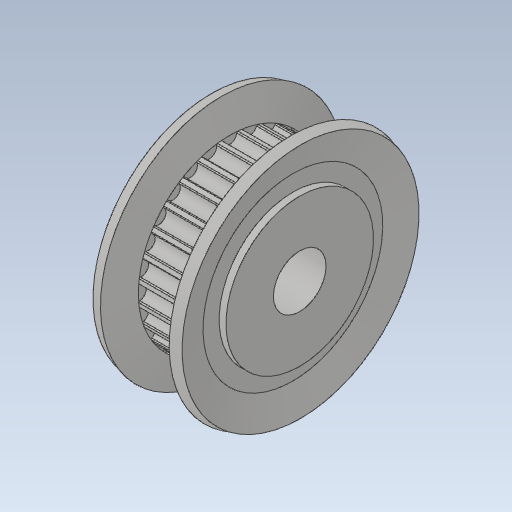
# Autodesk Inventor part: GPA28GT2040-A-H5_b
Saved by Autodesk Inventor 2024 (Build 280153000, 153)
## iProperties
Created: 2023-09-30
Part Number: GPA28GT2040-A-H5_b
Material: Generic
Catalog Web Link: www.cadenas.de
Description: GPA_GT2040, GPA_GT2060, GPA_GT2090, KGPA_GT2040, KGPA_GT2060, KGPA_GT2090, KGPK_GT2040, KGPK_GT2060, KGPK_GT2090_body-High Torque Timing Pulleys 2GT Type
Vendor: MISUMI
Document SubType Name: Modeling
Designer: psAdmin
Manufacturer: MISUMI
Mass: 1.92653 g
Surface Area: 18.9282 cm^2
Volume: 1.92653 cm^3
Density: 1 g/cm^3
Appearance: PSOLRGB-175-175-175
Category: PARTsolutions
Company: MISUMI
PSOL_IDENT_0: {$CADENAS_DATA/23d-libs/misumi/metric/51_timing_pulleys/gpa__gt2/gpa_gt2.prj},477 {VTYP=3D},{NB=GPA2
PSOL_IDENT_1: 8GT2040-A-H5_b},{LINA=GPA28GT2040-A-H5},{NN=GPA_GT2040, GPA_GT2060, GPA_GT2090, KGPA_GT2040, KGPA_GT
PSOL_IDENT_2: 2060, KGPA_GT2090, KGPK_GT2040, KGPK_GT2060, KGPK_GT2090_body},{DATE=25.04.2022 01:22:58},{GEOMDATE=
PSOL_IDENT_3: 22.12.2021 00:45:33},{VERSION=},{LINEID=100},{WBVAR=MAT,ST,TNW,PS,SBS,DD,Z,J,Q,R,S,T,ALT1,ALT2,M,QSC
PSOL_IDENT_4: ,QFC,QTC,ALT3,K,KSC,KFC,KTC,ALT4,ZM,ZSC,ZFC,ZTC,ALT5,BC,ALT6,ALT7,ALT8,FC,ALT13,BN},{WBNUMERIC=DD,Z,
PSOL_IDENT_5: J,Q,R,S,T,QSC,QFC,QTC,K,KSC,KFC,KTC,ZSC,ZFC,ZTC,BC,FC,BN}  {NB=GPA28GT2040-A-H5_b},{LINA=GPA28GT2040
PSOL_IDENT_6: -A-H5},{KT=DUMMY},{PN=GPA28GT2040-A-H5},{TYPE=GPA},{MAT=AA},{ST=CA},{NT=28},{TNW=GT2040},{BW=0},{A=5
PSOL_IDENT_7: .0},{W=8.3},{L=16.0},{PS=A},{PSA= 'A','B' },{SBS=H},{SBSALG= 'H','Round Hole','V','Stepped Hole' },{
PSOL_IDENT_8: DD=5.00},{DDALG=[5:6/1],[6.35],[7:10/1]},{DDHA=[5:6/1],[6.35],[7:10/1]},{DDHB=[5:6/1],[6.35],[7:8/1]
PSOL_IDENT_9: },{DDPA=},{DDPB=},{DDNA=},{DDNB=},{DDNKA=0},{DDNKB=0},{DDVA=[5:6/1],[6.35],[7:8/1]},{DDVFB=},{DDYA=[
PSOL_IDENT_10: 5:8/1]},{Z=0},{ZALG=0},{ZMIN=7},{ZAMAX=10},{ZBMAX=0},{J=0.0},{JALG=0},{JMAX=6.3},{Q=0},{R=0},{QRALG=
PSOL_IDENT_11: 0},{QRMIN=7},{QRMAX=10},{S=0.0},{SALG=0},{SMAX=2.300},{T=0.0},{TALG=0},{TMAX=5.000},{PD=17.83},{OD=1
PSOL_IDENT_12: 7.32},{D=10},{DE=14},{DDZ=5},{F=23},{E=14},{BB=0},{TT=0},{M1=3},{AC=-},{ALT1=},{ALT1A= '','Not appli
PSOL_IDENT_13: cable' },{ANG=115.714286},{ALT2=},{ALT2A= '','Not applicable' },{M=N/A},{MALG= 'N/A' },{MM=0.000},{M
PSOL_IDENT_14: PHD=0.000},{MA= 'N/A' },{MSA= 'N/A' },{QSC=0.0},{QSCA=0},{QFC=0.0},{QFCA=0},{QTC=0.0},{QTCA=0},{QPCD
PSOL_IDENT_15: MIN=9},{QPCDMINALG=9},{QPCDMAX=10},{ALT2PN=},{ALT3=},{ALT3A= '','Not applicable' },{K=0.0},{KA=0},{K
PSOL_IDENT_16: AMIN=4},{KAMAX=0},{KSMAX=0},{KSC=0.0},{KSCA=0},{KFC=0.0},{KFCA=0},{KTC=0.0},{KTCA=0},{KSCMIN=9.000},
PSOL_IDENT_17: {KPCDMIN=9.000},{KPCDMINALG=13.000},{KPCDMAX=10.000},{ALT3PN=},{ALT4=},{ALT4ALG= '','Not applicable'
PSOL_IDENT_18: },{ALT4MIN=15.500},{ALT4MAX=3.500},{ZM=N/A},{ZMALG= 'N/A' },{ZMFTALG= 'N/A' },{ZMSALG= 'N/A' },{ZMD
PSOL_IDENT_19: D1=0.0},{ZMDD2=0.0},{ZMHH=0.0},{ZSC=0.0},{ZSCALG=[0]},{ZFC=0.0},{ZFCALG=[0]},{ZTC=0.0},{ZTCALG=[0]},
PSOL_IDENT_20: {ZPCDMIN=0.000},{ZPCDMINALG=0.000},{ZPCDMAX=10.000},{ALT4PN=},{ALT5=},{ALT5ALG= '','Not applicable'
PSOL_IDENT_21: },{ALT5PN=},{BC=0.0},{BCALG=0},{BCMIN=3.000},{BCMAX=7.700},{ALT6=},{ALT7=},{ALT7ALG= '','w/o Flange
PSOL_IDENT_22: Attached on One Side Only','-RFC','with RFC (Flange Attached on The Boss Side Only)','-LFC','with LF
PSOL_IDENT_23: C (Flange Attached on The Opposite Side Only)' },{ALT8=},{ALT8ALG='','w/o FC (Flange Cut)','-FC','wi
PSOL_IDENT_24: th FC (Flange Cut)'},{ALT8PN=},{FC=0.0},{FCA=0},{ODAINT=20.500},{FCMIN=18.5},{FCMAX=21},{WLBC=8.3},{
PSOL_IDENT_25: SL=2.5},{SL2=2.5},{KTT=2.5},{KYY=6.16},{TAP=0},{MATALG= 'AA','Aluminum Alloy 2000 series' , '6000','
PSOL_IDENT_26: 6000 Series Aluminum Alloy' },{STALG= 'CA','Clear Anodize' },{ALT13=},{BN=0.000},{BNMIN=8.200},{BNMA
PSOL_IDENT_27: X=17.700},{ALT13ALG= '','Not applicable' },{BNALG=0},{BNPN=}
NB: GPA28GT2040-A-H5_b
NN: GPA_GT2040, GPA_GT2060, GPA_GT2090, KGPA_GT2040, KGPA_GT2060, KGPA_GT2090, KGPK_GT2040, KGPK_GT2060, KGPK_GT2090_body
NT: 28
NBSYN: $PN._b
LINA: GPA28GT2040-A-H5
CATALOG: Misumi
PN: GPA28GT2040-A-H5
MAT: Aluminum Alloy 2000 series
ST: Clear Anodize
TNW: GT2040
A: 5
W: 8.3
L: 16
PS: A
SBS: Round Hole
DD: 5
Z: 0
J: 0
Q: 0
R: 0
S: 0
T: 0
PD: 17.83
OD: 17.32
D: 10
F: 23
E: 14
AC: -
ALT1: Not applicable
ALT2: Not applicable
M: N/A
QSC: 0
QFC: 0
QTC: 0
ALT3: Not applicable
K: 0
KSC: 0
KFC: 0
KTC: 0
ALT4: Not applicable
ZM: N/A
ZMDD1: 0
ZMDD2: 0
ZMHH: 0
ZSC: 0
ZFC: 0
ZTC: 0
ALT5: Not applicable
BC: 0
ALT6: w/o Flange not Attached
ALT7: w/o Flange Attached on One Side Only
ALT8: w/o FC (Flange Cut)
FC: 0
ALT13: Not applicable
BN: 0
SUPPLIER: MISUMI
ARTICLENO: GPA28GT2040-A-H5_b
BOMINFO: GPA28GT2040-A-H5
CREATOR: CADENAS GmbH
Title: GPA28GT2040-A-H5
Author: Cadenas PARTsolutions
Comments: High Torque Timing Pulleys 2GT Type
Autodesk Inventor part; units mm, degrees
ref_plane "YZ Plane" through (0, 0, 0) normal (1, 0, 0) x (0, 1, 0)
ref_plane "XZ Plane" through (0, 0, 0) normal (0, 1, 0) x (-1, 0, 0)
ref_plane "XY Plane" through (0, 0, 0) normal (0, 0, 1) x (1, 0, 0)
sketch "Sketch_16" plane through (0, 0, 0) normal (0, 0, 1) x (1, 0, 0)
  line L0 (4.15, 0) -> (-4.15, 0)
  line L1 (-4.15, 0) -> (-4.15, 7)
  line L2 (-4.15, 7) -> (-2.5, 7)
  line L3 (-2.5, 7) -> (-2.5, 8.66)
  line L4 (-2.5, 8.66) -> (2.5, 8.66)
  line L5 (2.5, 8.66) -> (2.5, 7)
  line L6 (2.5, 7) -> (4.15, 7)
  line L7 (4.15, 7) -> (4.15, 0)
  line L8 (4.15, 0) -> (-4.15, 0)
  constraints: 18 end point
revolve "Revolution1" add sketch "Sketch_16" angle 360 about axis through (4.15, 0, 0) along (1, 0, 0)
sketch "Sketch_18" plane through (0, 0, 0) normal (1, 0, 0) x (0, 1, 0)
  line L0 (8.8642, 0.9508) -> (8.6126, 0.9238)
  line L1 (8.6126, 0.9238) -> (8.6245, 0.7939)
  arc A0 (8.5234, 0.6721) -> (8.6245, 0.7939) centre (8.513, 0.7836) ccw
  arc A1 (8.5234, 0.6721) -> (8.5234, -0.6721) centre (8.586, 0) ccw
  arc A2 (8.6245, -0.7939) -> (8.5234, -0.6721) centre (8.513, -0.7836) ccw
  line L2 (8.6245, -0.7939) -> (8.6126, -0.9238)
  line L3 (8.6126, -0.9238) -> (8.8642, -0.9508)
  arc A3 (8.8642, -0.9508) -> (8.8642, 0.9508) centre (0, 0) ccw
  constraints: 8 end point, 8 point on circle, 4 centre point
extrude "Extrusion1" cut sketch "Sketch_18" along normal mid plane 5
pattern_circular "Circular Pattern1" count 28 over 360 about axis through (0, 0, 0) along (1, 0, 0) of "Extrusion1"
sketch "Sketch_20" plane through (0, 0, 0) normal (0, 0, 1) x (1, 0, 0)
  line L0 (50, 0) -> (-50, 0)
  line L1 (2.5, 8.66) -> (2.5, 7)
  line L2 (2.5, 7) -> (3.5, 7)
  line L3 (3.5, 7) -> (3.5, 8.5283)
  line L4 (3.5, 8.5283) -> (4.2269, 11.2412)
  line L5 (4.2269, 11.2412) -> (3.261, 11.5)
  line L6 (3.261, 11.5) -> (2.5, 8.66)
  constraints: 14 end point
revolve "Revolution2" add sketch "Sketch_20" angle 360 about axis through (50, 0, 0) along (1, 0, 0)
sketch "Sketch_21" plane through (0, 0, 0) normal (0, 0, 1) x (1, 0, 0)
  line L0 (50, 0) -> (-50, 0)
  line L1 (-4.2269, 11.2412) -> (-3.5, 8.5283)
  line L2 (-3.5, 8.5283) -> (-3.5, 7)
  line L3 (-3.5, 7) -> (-2.5, 7)
  line L4 (-2.5, 7) -> (-2.5, 8.66)
  line L5 (-2.5, 8.66) -> (-3.261, 11.5)
  line L6 (-3.261, 11.5) -> (-4.2269, 11.2412)
  constraints: 14 end point
revolve "Revolution3" add sketch "Sketch_21" angle 360 about axis through (50, 0, 0) along (1, 0, 0)
sketch "Sketch5" plane through (4.15, 0, 0) normal (1, 0, 0) x (0, 0, -1)
  point P0 (0, 0)
hole "Hole1" at (4.15, 0, 0) direction (-1, 0, 0) diameter 5 depth 8.3
body "Solid1"
